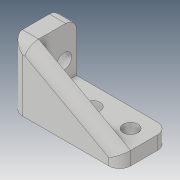
# Autodesk Inventor part: servoMount
Saved by Autodesk Inventor 2018 (Build 220112000, 112)
## iProperties
Created: 2020-01-20
Part Number: servoMount
Material: Generic
Document SubType Name: Modeling
Designer: anirudh
Density: 1 g/cm^3
Appearance: Default
Author: anirudh
Autodesk Inventor part; units mm, degrees
ref_plane "YZ Plane" through (0, 0, 0) normal (1, 0, 0) x (0, 1, 0)
ref_plane "XZ Plane" through (0, 0, 0) normal (0, 1, 0) x (-1, 0, 0)
ref_plane "XY Plane" through (0, 0, 0) normal (0, 0, 1) x (1, 0, 0)
sketch "Sketch1" plane through (0, 0, 0) normal (0, 1, 0) x (-1, 0, 0)
  line L0 (0, 0) -> (-25.4, 0)
  line L1 (-25.4, 0) -> (-25.4, 8.89)
  line L2 (-25.4, 8.89) -> (0, 8.89)
  line L3 (0, 8.89) -> (0, 0)
  dimension "d0" = 25.4
  dimension "d1" = 8.89
  constraints: 8 end point, 2 parallel, 1 horizontal, 1 perpendicular
  measures "d0" distance of L1.end L2.end
  measures "d1" distance of L0.end L1.end
extrude "Extrusion1" add sketch "Sketch1" along normal blind 3.81
sketch "Sketch2" plane through (0, 3.81, 0) normal (0, 1, 0) x (1, 0, 0)
  line L0 (0, -8.89) -> (25.4, -8.89) projected
  line L1 (0, 0) -> (3.81, 0)
  line L2 (3.81, 0) -> (3.81, -8.89)
  line L3 (3.81, -8.89) -> (0, -8.89)
  line L4 (0, -8.89) -> (0, 0)
  dimension "d4" = 3.81
  constraints: 8 end point, 2 parallel, 1 horizontal, 1 perpendicular, 1 point on line
  measures "d4" distance of L2.end L3.end
extrude "Extrusion2" add sketch "Sketch2" along normal blind 11.2014
sketch "Sketch3" plane through (0, 0, 0) normal (-1, 0, 0) x (0, 0, 1)
  arc A0 (2.8956, 9.2557) -> (2.8956, 5.7557) centre (2.8956, 7.5057) ccw
  circle A1 centre (2.8956, 7.5057) radius 1.75
  point P0 (0, 0)
  point P1 (0, 15.0114)
  constraints: 2 point on circle, 1 centre point, 1 coincident, 1 vertical alignment, 2 other
extrude "Extrusion3" cut sketch "Sketch3" against normal blind 11.2014
sketch "Sketch4" plane through (0, 0, 8.89) normal (0, 0, 1) x (1, 0, 0)
  line L0 (3.81, 3.81) -> (25.4, 3.81) projected
  line L1 (25.4, 3.81) -> (3.81, 3.81)
  line L2 (3.81, 3.81) -> (3.81, 3.175)
  line L3 (3.81, 3.175) -> (25.4, 3.175)
  line L4 (25.4, 3.175) -> (25.4, 3.81)
  point P0 (0, 0)
  dimension "d11" = 0.635
  constraints: 8 end point, 2 parallel, 1 horizontal, 1 perpendicular
  measures "d11" distance of L2.end L1.end
extrude "Extrusion4" cut sketch "Sketch4" against normal blind 11.2014
sketch "Sketch5" plane through (3.81, 3.175, 8.89) normal (0, 1, 0) x (1, 0, 0)
  line L0 (12.7, 0) -> (3.81, 0)
  circle A0 centre (8.255, 4.445) radius 1.75
  circle A1 centre (17.145, 4.445) radius 1.75
  point P0 (21.59, 8.89)
  dimension "d16" = 3.5
  dimension "d17" = 3.5
  constraints: 2 centre point, 2 end point, 1 horizontal
  measures "d16" diameter of A0
  measures "d17" diameter of A1
extrude "Extrusion5" cut sketch "Sketch5" against normal blind 11.2014
sketch "Sketch6" plane through (0, 0, 8.89) normal (0, 0, 1) x (1, 0, 0)
  line L0 (0, 15.0114) -> (3.81, 15.0114) projected
  line L1 (3.81, 15.0114) -> (0, 15.0114)
  line L2 (0, 15.0114) -> (0, 0)
  line L3 (25.4, 0) -> (25.4, 3.175) projected
  line L4 (0, 0) -> (25.4, 0)
  line L5 (25.4, 0) -> (25.4, 3.175)
  line L6 (25.4, 3.175) -> (3.81, 15.0114)
  constraints: 10 end point, 3 perpendicular, 1 horizontal
extrude "Extrusion6" add sketch "Sketch6" along normal blind 2.54
fillet "Fillet1" radius 2.54 6 edges at (0, 7.5057, 11.43) (14.605, 9.0932, 11.43) (25.4, 1.5875, 11.43) (25.4, 1.5875, 0) (1.905, 15.0114, 0) (1.905, 15.0114, 11.43)
body "Solid1"
